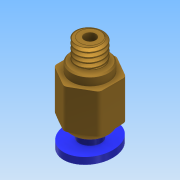
# Autodesk Inventor part: fitting
Saved by Autodesk Inventor 2017 (Build 210142000, 142)
## iProperties
Part Number: fitting
Material: Типовые
Document SubType Name: Modeling
Designer: STALKER
Density: 1 g/cm^3
Appearance: Латунь - сатинированная
Author: STALKER
Autodesk Inventor part; units mm, degrees
ref_plane "YZ Plane" through (0, 0, 0) normal (1, 0, 0) x (0, 1, 0)
ref_plane "XZ Plane" through (0, 0, 0) normal (0, 1, 0) x (-1, 0, 0)
ref_plane "XY Plane" through (0, 0, 0) normal (0, 0, 1) x (1, 0, 0)
sketch "Эскиз1" plane through (0, 0, 0) normal (0, 0, 1) x (1, 0, 0)
  line L0 (0, 0) -> (0, 11.4297) construction
  line L1 (0, 0) -> (-16, 0) construction
  line L2 (0, 5.7735) -> (5, 2.8868)
  line L3 (5, 2.8868) -> (5, -2.8868)
  line L4 (5, -2.8868) -> (0, -5.7735)
  line L5 (0, -5.7735) -> (-5, -2.8868)
  line L6 (-5, -2.8868) -> (-5, 2.8868)
  line L7 (-5, 2.8868) -> (0, 5.7735)
  circle A0 centre (0, 0) radius 4.5
  circle A1 centre (0, 0) radius 3
  circle A2 centre (0, 0) radius 2.1
  circle A3 centre (0, 0) radius 4.1
  circle A4 centre (0, 0) radius 1.25
  dimension "d0" = 10
  dimension "d1" = 9
  dimension "d2" = 6
  dimension "d3" = 4.2
  dimension "d4" = 8.2
  dimension "d5" = 2.5
  constraints: 16 end point, 6 coincident, 5 centre point, 1 horizontal, 1 point on line, 13 other
  measures "d0" distance between parallel lines of L6 L3
  measures "d1" diameter of A0
  measures "d2" diameter of A1
  measures "d3" diameter of A2
  measures "d4" diameter of A3
  measures "d5" diameter of A4
extrude "Выдавливание1" add sketch "Эскиз1" along normal blind 6.5 contours A1 | A2
extrude "Выдавливание2" add sketch "Эскиз1" along normal blind 2 contours A1 | A3
extrude "Выдавливание3" add sketch "Эскиз1" against normal blind 14 contours A2
extrude "Выдавливание4" add sketch "Эскиз1" against normal blind 8.8 contours L2 L3 L4 L5 L6 L7 | A0 | A1 | A3
extrude "Выдавливание5" add sketch "Эскиз1" against normal blind 10.8 contours A0 | A1 | A2 | A3
fillet "Сопряжение1" radius 2 1 edges at (-4.5, 0, -10.8)
fillet "Сопряжение2" radius 1 6 edges at (5, 2.8868, -4.4) (0, 5.7735, -4.4) (5, -2.8868, -4.4) (0, -5.7735, -4.4) (-5, -2.8868, -4.4) (-5, 2.8868, -4.4)
sketch "Эскиз2" plane through (0, 0, 0) normal (1, 0, 0) x (0, 1, 0)
  line L0 (0, 0) -> (0, -22) construction
  line L1 (6, -8.5) -> (4.5, -8.8)
  line L2 (4.5, -8.8) -> (6.1646, -9.323)
  line L3 (6.1646, -9.323) -> (6, -8.5)
  line L4 (4.5, -8.8) -> (-4.5, -8.8) projected
  line L5 (2.5, -10.8) -> (-2.5, -10.8) projected
  line L6 (3.1754, -8.8) -> (5.4848, -8.8) projected
  dimension "d18" = 0.3
  constraints: 8 end point, 1 perpendicular, 1 vertical
  measures "d18" distance from line of L1.start L6
revolve "Вращение1" cut sketch "Эскиз2" angle 360 about axis through (0, 0, 0) along (0, 0, -1)
sketch "Эскиз3" plane through (0, 0, -10.8) normal (0, 0, -1) x (-1, 0, 0)
  circle A0 centre (0, 0) radius 2.5
  circle A1 centre (0, 0) radius 2.4
  circle A2 centre (0, 0) radius 2.1
  dimension "d20" = 5
  dimension "d21" = 0.1
  dimension "d22" = 4.2
  constraints: 3 centre point, 3 coincident
  measures "d20" diameter of A0
  measures "d21" radial gap between concentric circles of A0 A1
  measures "d22" diameter of A2
extrude "Выдавливание6" cut sketch "Эскиз3" against normal blind 5 contours A0
sketch "Эскиз4" plane through (0, 0, -14) normal (0, 0, -1) x (-1, 0, 0)
  ellipse E0 centre (0, 0) end of major axis (0, 5.8) minor radius 5
  dimension "d25" = 5.8
  dimension "d26" = 5
  constraints: 1 coincident, 2 other
extrude "Выдавливание7" add sketch "Эскиз4" against normal blind 1.5
extrude "Выдавливание8" cut sketch "Эскиз3" along normal mid plane 10 contours A2
chamfer "Фаска1" distance 0.3 angle 45 1 edges at (-4.1, 0, 2)
sketch "Эскиз5" plane through (0, 0, -10.8) normal (0, 0, -1) x (-1, 0, 0)
  circle A0 centre (0, 0) radius 2.4 projected
  circle A1 centre (0, 0) radius 2.1 projected
extrude "Выдавливание9" add sketch "Эскиз5" along normal blind 2
thread "Резьба1" size "M6x1" class "6g" standard "ANSI Metric M Profile" full length
sketch "Эскиз7" plane through (0, 0, 6.5) normal (-1, 0, 0) x (0, 1, 0)
  line L0 (3, 0) -> (3, 4.5)
  line L1 (3, 4.5) -> (2.2585, 4.5)
  line L2 (2.2585, 4.5) -> (2.2585, 0)
  line L3 (2.2585, 0) -> (3, 0)
  line L4 (0, -5.4086) -> (0, 24.8181) projected
  constraints: 8 end point
revolve "Вращение2" cut sketch "Эскиз7" angle 360 about axis through (0, 0, 6.5) along (0, 0, -1)
sketch "Эскиз8" plane through (0, 0, 6.5) normal (-1, 0, 0) x (0, 1, 0)
  line L0 (3, 0) -> (3, 4.5)
  line L1 (3, 4.5) -> (2.2585, 4.5)
  line L2 (2.2585, 4.5) -> (2.2585, 0)
  line L3 (2.2585, 0) -> (3, 0)
  line L4 (0, -5.4086) -> (0, 24.8181) projected
  constraints: 8 end point
revolve "Вращение3" add sketch "Эскиз8" angle 360 about axis through (0, 0, 6.5) along (0, 0, -1) separate body
sketch "Эскиз6" plane through (0, 0, 6.5) normal (1, 0, 0) x (0, 0, -1)
  line L0 (-0.5834, -2.3093) -> (-0.5001, -2.3093) construction
  line L1 (0.0832, -2.9496) -> (-0.0001, -3.1097) construction
  line L2 (-1.0001, -3.1097) -> (-1.0834, -2.9496) construction
  line L3 (-0.4168, -2.3093) -> (-0.5001, -2.1492) construction
  line L4 (-0.5001, -2.1492) -> (-0.5834, -2.3093) construction
  line L5 (-1.0001, -3.1097) -> (-0.9168, -2.9496) construction
  line L6 (-0.4168, -2.3093) -> (-0.0834, -2.9496)
  line L7 (-1.0834, -2.9496) -> (-0.9168, -2.9496) construction
  arc A0 (-1.0834, -2.9496) -> (-1.0001, -3.0002) centre (-1.0001, -2.9062) ccw construction
  line L8 (0.0832, -2.9496) -> (-0.0834, -2.9496) construction
  line L9 (-1.0001, -3.1097) -> (-1.0001, -2.9496) construction
  line L10 (-0.0001, -3.1097) -> (-0.0001, -2.9496) construction
  line L11 (-0.5001, -2.1492) -> (-0.5001, -2.2587) construction
  line L12 (-1.0001, -3.0002) -> (-0.0001, -3.0002)
  arc A1 (-1.0001, -3.0002) -> (-0.9168, -2.9496) centre (-1.0001, -2.9062) ccw
  line L13 (-0.0834, -2.9496) -> (-0.0001, -3.1097) construction
  line L14 (-0.9168, -2.9496) -> (-0.5834, -2.3093)
  line L15 (-0.0001, -0.0002) -> (-0.0001, 0.0177)
  line L16 (-0.0001, 0.0177) -> (-0.0001, -0.0002)
  line L17 (-0.0001, -0.0002) -> (0.0334, -0.0002)
  arc A2 (-0.0834, -2.9496) -> (-0.0001, -3.0002) centre (-0.0001, -2.9062) ccw
  arc A3 (-0.0001, -3.0002) -> (0.0832, -2.9496) centre (-0.0001, -2.9062) ccw construction
  arc A4 (-0.5001, -2.2587) -> (-0.5834, -2.3093) centre (-0.5001, -2.3527) ccw
  arc A5 (-0.4168, -2.3093) -> (-0.5001, -2.2587) centre (-0.5001, -2.3527) ccw
  line L18 (-0.5001, -2.2587) -> (-0.5001, -2.3093) construction
  line L19 (-0.5001, -2.3093) -> (-0.4168, -2.3093) construction
  dimension "d38" = 55
  dimension "d39" = 0.1601
  dimension "d40" = 0.1601
  dimension "Эскиз6_ThreadOffset" = 0
  dimension "Эскиз6_MajorRadius" = 3
  dimension "d43" = 1
  dimension "Эскиз6_MinorRadius" = 2.2585
  constraints: 40 end point, 12 point on circle, 10 parallel, 8 tangent, 6 centre point, 6 collinear, 2 midpoint, 2 point on line, 1 horizontal, 1 perpendicular, 3 other
  measures "d38" angle of L6 L14
  measures "d39" distance of L3.end L0.end
  measures "d40" distance of L1.end L10.end
  measures "Эскиз6_ThreadOffset" distance between parallel lines of L15 L10
  measures "Эскиз6_MajorRadius" distance from line of L12 L15.start
  measures "d43" distance from line of L1.end L9
  measures "Эскиз6_MinorRadius" distance edge to line of A5 L17
coil "Пружина1" sketch "Эскиз6" operation cut axis through (0, 0, 6.5) along (0, 0, -1) pitch 1.001 turns 6.493506 hand right bodies 2
equation "\"d38\" = d45"
equation "\"d39\" = 0.160083 * Эскиз6_Pitch"
equation "\"d40\" = 0.160083 * Эскиз6_Pitch"
equation "\"d43\" = Эскиз6_Pitch"
equation "\"d45\" = 55deg"
equation "\"Эскиз6_Pitch\" = 1"
